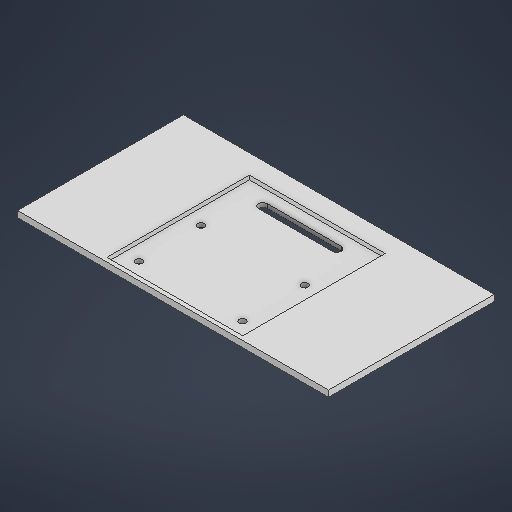
# Autodesk Inventor part: TOPLeft
Saved by Autodesk Inventor 2026.1 (Build 301233020, 233B)
## iProperties
Created: 2026-07-07
Part Number: TOPLeft
Material: Generic
Document SubType Name: Modeling
Designer: pleased
Density: 1 g/cm^3
Appearance: Default
Author: pleased
Autodesk Inventor part; units mm, degrees
ref_plane "YZ Plane" through (0, 0, 0) normal (1, 0, 0) x (0, 1, 0)
ref_plane "XZ Plane" through (0, 0, 0) normal (0, 1, 0) x (-1, 0, 0)
ref_plane "XY Plane" through (0, 0, 0) normal (0, 0, 1) x (1, 0, 0)
sketch "Sketch1" plane through (0, 0, 0) normal (0, 1, 0) x (-1, 0, 0)
  line L0 (0, 80) -> (150, 80)
  line L1 (150, 80) -> (150, 0)
  line L2 (150, 0) -> (0, 0)
  line L3 (0, 0) -> (0, 80)
  point P0 (0, 0)
  dimension "d0" = 150
  dimension "d1" = 80
  constraints: 8 end point, 2 parallel, 1 horizontal, 1 perpendicular
  measures "d0" distance of L1.end L2.end
  measures "d1" distance of L0.end L1.end
extrude "Extrusion1" add sketch "Sketch1" along normal blind 3
sketch "Sketch2" plane through (0, 3, 0) normal (0, 1, 0) x (1, 0, 0)
  line L0 (-93.7, -18) -> (-58, -18)
  line L1 (-93.7, -18) -> (-58, -18) construction
  line L2 (-93.7, -20.1) -> (-58, -20.1)
  line L3 (-58, -15.9) -> (-93.7, -15.9)
  arc A0 (-93.7, -15.9) -> (-93.7, -20.1) centre (-93.7, -18) ccw
  arc A1 (-58, -20.1) -> (-58, -15.9) centre (-58, -18) ccw
  circle A2 centre (-100.5, -71) radius 1.65
  circle A3 centre (-100.5, -41) radius 1.65
  circle A4 centre (-50.5, -71) radius 1.65
  circle A5 centre (-50.5, -41) radius 1.65
  point P0 (0, 0)
  point P1 (-50.5, -18)
  point P2 (-92, -41)
  point P3 (-92, -71)
  point P4 (-75.85, -18)
  dimension "d4" = 4.2
  dimension "d5" = 3.3
  dimension "d6" = 3.3
  dimension "d7" = 3.3
  dimension "d8" = 3.3
  constraints: 10 end point, 6 centre point, 4 coincident, 4 point on circle, 4 tangent, 2 equal length, 1 horizontal, 1 midpoint
  measures "d4" diameter of A1
  measures "d5" diameter of A2
  measures "d6" diameter of A3
  measures "d7" diameter of A4
  measures "d8" diameter of A5
extrude "Extrusion2" cut sketch "Sketch2" against normal blind 3
sketch "Sketch3" plane through (0, 3, 0) normal (0, 1, 0) x (1, 0, 0)
  line L0 (-107.9014, -77.0296) -> (-44.3595, -77.0296)
  line L1 (-44.3595, -77.0296) -> (-44.3595, -10.2906)
  line L2 (-44.3595, -10.2906) -> (-107.9014, -10.2906)
  line L3 (-107.9014, -10.2906) -> (-107.9014, -77.0296)
  point P0 (0, 0)
  constraints: 8 end point, 2 parallel, 1 horizontal, 1 perpendicular
extrude "Extrusion3" cut sketch "Sketch3" against normal blind 1
chamfer "Chamfer1" distance 1 angle 45 4 edges at (-107.9014, 3, 43.6601) (-76.1304, 3, 10.2906) (-44.3595, 3, 43.6601) (-76.1304, 3, 77.0296)
body "Solid1"
